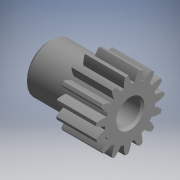
# Autodesk Inventor part: PS1-15_On
Saved by Autodesk Inventor 2017.3 (Build 213256000, 256)
## iProperties
Part Number: PS1-15_On
Material: Generic
Catalog Web Link: www.cadenas.de
Description: Plastic Spur Gears (PS)-
Vendor: KHK
Document SubType Name: Modeling
Designer: partserver
Manufacturer: KHK
Mass: 2.26777 g
Surface Area: 19.5536 cm^2
Volume: 2.26777 cm^3
Density: 1 g/cm^3
Appearance: PSOLRGB-175-175-175
Category: PARTsolutions
Company: KHK
Title: PS1-15
Author: Cadenas PARTsolutions
PSOL_IDENT_0: {$CADENAS_DATA\23d-libs\khk\spur_gears\plastic_spur_gears_ps.prj},177 {VTYP=3D},{NB=PS1-15_On},{LINA=
PSOL_IDENT_1: PS1-15},{NN=Plastic Spur Gears (PS)},{DATE=10.04.2020 06:07:24},{GEOMDATE=05.07.2019 08:26:52},{VERS
PSOL_IDENT_2: ION=},{LINEID=20},{WBVAR=TOOTH},{WBNUMERIC=}  {NB=PS1-15_On},{LINA=PS1-15},{KT=DUMMY},{CN=PS1-15},{M=
PSOL_IDENT_3: 1},{MX=1.000},{Z=15},{S=S1},{A=6},{B=12},{C=15.0},{D=17.0},{E=10},{F=10},{G=20},{K=0},{KD=0.0},{M1=0
PSOL_IDENT_4: },{SCSX=0},{J=0.0},{WMF=S1003.WMF},{R=0.2},{N=0.5},{L=0.1},{L2=0.5},{CBD1=0.0},{CBD2=0.0},{TOOTH=On}
NB: PS1-15_On
NN: Plastic Spur Gears (PS)
NBSYN: $CN._$TOOTH.
LINA: PS1-15
CATALOG: KHK
CN: PS1-15
M: 1
Z: 15
S: S1
A: 6
B: 12
C: 15
D: 17
E: 10
F: 10
G: 20
K: 0
KD: 0
M1: 0
J: 0
TOOTH: On
SUPPLIER: KHK
ARTICLENO: PS1-15_On
BOMINFO: PS1-15
CREATOR: CADENAS GmbH
Autodesk Inventor part; units mm, degrees
ref_plane "YZ Plane" through (0, 0, 0) normal (1, 0, 0) x (0, 1, 0)
ref_plane "XZ Plane" through (0, 0, 0) normal (0, 1, 0) x (-1, 0, 0)
ref_plane "XY Plane" through (0, 0, 0) normal (0, 0, 1) x (1, 0, 0)
sketch "Sketch_8" plane through (0, 0, 0) normal (0, 0, 1) x (1, 0, 0)
  line L0 (20, 0) -> (0, 0)
  line L1 (0, 3.5) -> (0.5, 3)
  line L2 (0.5, 3) -> (19.5, 3)
  line L3 (19.5, 3) -> (20, 3.5)
  line L4 (20, 3.5) -> (20, 5.5)
  line L5 (20, 5.5) -> (19.5, 6)
  line L6 (19.5, 6) -> (10.2, 6)
  arc A0 (10, 6.2) -> (10.2, 6) centre (10.2, 6.2) ccw
  line L7 (10, 6.2) -> (10, 8.4)
  line L8 (10, 8.4) -> (9.9, 8.5)
  line L9 (9.9, 8.5) -> (0.1, 8.5)
  line L10 (0.1, 8.5) -> (0, 8.4)
  line L11 (0, 8.4) -> (0, 3.5)
  constraints: 24 end point, 2 point on circle, 1 centre point
revolve "Revolution1" add sketch "Sketch_8" angle 360 about axis through (20, 0, 0) along (1, 0, 0)
sketch "Sketch_11" plane through (0, 0, 0) normal (1, 0, 0) x (0, 1, 0)
  line L0 (17, 17) -> (-17, 17)
  line L1 (-17, 17) -> (-17, -17)
  line L2 (-17, -17) -> (17, -17)
  line L3 (17, -17) -> (17, 17)
  arc A0 (-0.5337, 8.4832) -> (-1.2417, 8.4088) centre (0, 0) ccw
  arc A1 (-1.2417, 8.4088) -> (-1.5543, 6.0536) centre (4.4321, 6.4574) ccw
  arc A2 (-1.5543, 6.0536) -> (-2.3008, 5.8111) centre (0, 0) ccw
  arc A3 (-2.3008, 5.8111) -> (-3.938, 7.5327) centre (-7.3812, 2.619) ccw
  arc A4 (-3.938, 7.5327) -> (-4.5545, 7.1768) centre (0, 0) ccw
  arc A5 (-4.5545, 7.1768) -> (-3.8822, 4.8981) centre (1.4225, 7.7018) ccw
  arc A6 (-3.8822, 4.8981) -> (-4.4655, 4.3729) centre (0, 0) ccw
  arc A7 (-4.4655, 4.3729) -> (-6.6614, 5.2798) centre (-7.8083, -0.6096) ccw
  arc A8 (-6.6614, 5.2798) -> (-7.0798, 4.7038) centre (0, 0) ccw
  arc A9 (-7.0798, 4.7038) -> (-5.5388, 2.8956) centre (-1.8331, 7.6145) ccw
  arc A10 (-5.5388, 2.8956) -> (-5.858, 2.1786) centre (0, 0) ccw
  arc A11 (-5.858, 2.1786) -> (-8.233, 2.1139) centre (-6.8853, -3.7328) ccw
  arc A12 (-8.233, 2.1139) -> (-8.381, 1.4175) centre (0, 0) ccw
  arc A13 (-8.381, 1.4175) -> (-6.2377, 0.3924) centre (-4.7718, 6.2106) ccw
  arc A14 (-6.2377, 0.3924) -> (-6.2377, -0.3924) centre (0, 0) ccw
  arc A15 (-6.2377, -0.3924) -> (-8.381, -1.4175) centre (-4.7718, -6.2106) ccw
  arc A16 (-8.381, -1.4175) -> (-8.233, -2.1139) centre (0, 0) ccw
  arc A17 (-8.233, -2.1139) -> (-5.858, -2.1786) centre (-6.8853, 3.7328) ccw
  arc A18 (-5.858, -2.1786) -> (-5.5388, -2.8956) centre (0, 0) ccw
  arc A19 (-5.5388, -2.8956) -> (-7.0798, -4.7038) centre (-1.8331, -7.6145) ccw
  arc A20 (-7.0798, -4.7038) -> (-6.6614, -5.2798) centre (0, 0) ccw
  arc A21 (-6.6614, -5.2798) -> (-4.4655, -4.3729) centre (-7.8083, 0.6096) ccw
  arc A22 (-4.4655, -4.3729) -> (-3.8822, -4.8981) centre (0, 0) ccw
  arc A23 (-3.8822, -4.8981) -> (-4.5545, -7.1768) centre (1.4225, -7.7018) ccw
  arc A24 (-4.5545, -7.1768) -> (-3.938, -7.5327) centre (0, 0) ccw
  arc A25 (-3.938, -7.5327) -> (-2.3008, -5.8111) centre (-7.3812, -2.619) ccw
  arc A26 (-2.3008, -5.8111) -> (-1.5543, -6.0536) centre (0, 0) ccw
  arc A27 (-1.5543, -6.0536) -> (-1.2417, -8.4088) centre (4.4321, -6.4574) ccw
  arc A28 (-1.2417, -8.4088) -> (-0.5337, -8.4832) centre (0, 0) ccw
  arc A29 (-0.5337, -8.4832) -> (0.2617, -6.2445) centre (-5.6778, -5.3948) ccw
  arc A30 (0.2617, -6.2445) -> (1.0423, -6.1625) centre (0, 0) ccw
  arc A31 (1.0423, -6.1625) -> (2.2858, -8.1869) centre (6.6754, -4.0964) ccw
  arc A32 (2.2858, -8.1869) -> (2.9629, -7.9669) centre (0, 0) ccw
  arc A33 (2.9629, -7.9669) -> (2.779, -5.5982) centre (-2.9927, -7.2378) ccw
  arc A34 (2.779, -5.5982) -> (3.4587, -5.2058) centre (0, 0) ccw
  arc A35 (3.4587, -5.2058) -> (5.4181, -6.5494) centre (7.7644, -1.0272) ccw
  arc A36 (5.4181, -6.5494) -> (5.9471, -6.073) centre (0, 0) ccw
  arc A37 (5.9471, -6.073) -> (4.8157, -3.9839) centre (0.2099, -7.8293) ccw
  arc A38 (4.8157, -3.9839) -> (5.277, -3.3489) centre (0, 0) ccw
  arc A39 (5.277, -3.3489) -> (7.6135, -3.7794) centre (7.5109, 2.2197) ccw
  arc A40 (7.6135, -3.7794) -> (7.9031, -3.1291) centre (0, 0) ccw
  arc A41 (7.9031, -3.1291) -> (6.0198, -1.6807) centre (3.3762, -7.067) ccw
  arc A42 (6.0198, -1.6807) -> (6.183, -0.913) centre (0, 0) ccw
  arc A43 (6.183, -0.913) -> (8.4925, -0.3559) centre (5.9587, 5.0828) ccw
  arc A44 (8.4925, -0.3559) -> (8.4925, 0.3559) centre (0, 0) ccw
  arc A45 (8.4925, 0.3559) -> (6.183, 0.913) centre (5.9587, -5.0828) ccw
  arc A46 (6.183, 0.913) -> (6.0198, 1.6807) centre (0, 0) ccw
  arc A47 (6.0198, 1.6807) -> (7.9031, 3.1291) centre (3.3762, 7.067) ccw
  arc A48 (7.9031, 3.1291) -> (7.6135, 3.7794) centre (0, 0) ccw
  arc A49 (7.6135, 3.7794) -> (5.277, 3.3489) centre (7.5109, -2.2197) ccw
  arc A50 (5.277, 3.3489) -> (4.8157, 3.9839) centre (0, 0) ccw
  arc A51 (4.8157, 3.9839) -> (5.9471, 6.073) centre (0.2099, 7.8293) ccw
  arc A52 (5.9471, 6.073) -> (5.4181, 6.5494) centre (0, 0) ccw
  arc A53 (5.4181, 6.5494) -> (3.4587, 5.2058) centre (7.7644, 1.0272) ccw
  arc A54 (3.4587, 5.2058) -> (2.779, 5.5982) centre (0, 0) ccw
  arc A55 (2.779, 5.5982) -> (2.9629, 7.9669) centre (-2.9927, 7.2378) ccw
  arc A56 (2.9629, 7.9669) -> (2.2858, 8.1869) centre (0, 0) ccw
  arc A57 (2.2858, 8.1869) -> (1.0423, 6.1625) centre (6.6754, 4.0964) ccw
  arc A58 (1.0423, 6.1625) -> (0.2617, 6.2445) centre (0, 0) ccw
  arc A59 (0.2617, 6.2445) -> (-0.5337, 8.4832) centre (-5.6778, 5.3948) ccw
  constraints: 120 point on circle, 60 centre point, 8 end point
extrude "Extrusion1" cut sketch "Sketch_11" along normal blind 10
body "Solid1"
